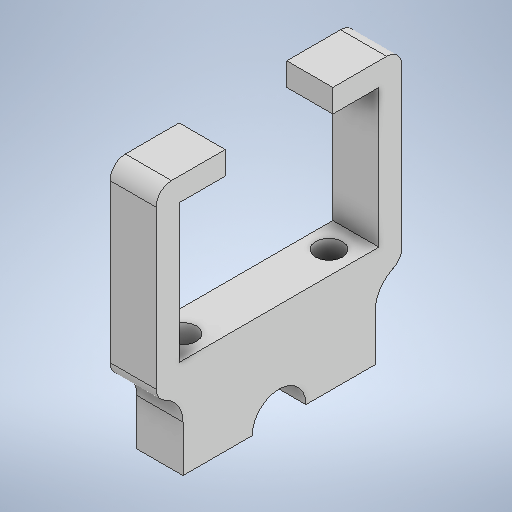
# Autodesk Inventor part: Base
Saved by Autodesk Inventor 2025 (Build 290162000, 162)
## iProperties
Created: 2024-06-05
Part Number: Base
Material: Générique
Document SubType Name: Modeling
Designer: luc4s
Density: 1 g/cm^3
Appearance: Par défaut
Author: luc4s
## iProperties of the stored document Bras_1_Impression 3D.ipt
Created: 2024-06-05
Part Number: Bras_1_Impression 3D
Material: Générique
Document SubType Name: Modeling
Designer: luc4s
Density: 1 g/cm^3
Appearance: Par défaut
Author: luc4s
Autodesk Inventor part; units mm, degrees
ref_plane "YZ Plane" through (0, 0, 0) normal (1, 0, 0) x (0, 1, 0)
ref_plane "XZ Plane" through (0, 0, 0) normal (0, 1, 0) x (-1, 0, 0)
ref_plane "XY Plane" through (0, 0, 0) normal (0, 0, 1) x (1, 0, 0)
sketch "Esquisse1" plane through (0, 0, 0) normal (1, 0, 0) x (0, 1, 0)
  arc A0 (0, -3.5) -> (0, 3.5) centre (0, 0) ccw
  line L0 (0, 6.2947) -> (0, -6.5718) construction
  line L1 (0, 3.5) -> (0, 12.5)
  line L2 (0, 12.5) -> (10, 12.5)
  line L3 (10, -12.5) -> (0, -12.5)
  line L4 (0, -12.5) -> (0, -3.5)
  line L5 (10, 12.5) -> (10, 16)
  line L6 (10, 16) -> (34, 16)
  line L7 (34, 16) -> (34, 7)
  line L8 (34, 7) -> (31, 7)
  line L9 (31, 7) -> (31, 13)
  line L10 (31, 13) -> (13, 13)
  line L11 (13, 13) -> (13, -13)
  line L12 (13, -13) -> (31, -13)
  line L13 (31, -13) -> (31, -7)
  line L14 (31, -7) -> (34, -7)
  line L15 (34, -7) -> (34, -16)
  line L16 (34, -16) -> (10, -16)
  line L17 (10, -16) -> (10, -12.5)
  point P0 (22, 13)
  dimension "d16" = 3.5
  dimension "d17" = 25
  dimension "d18" = 26
  dimension "d19" = 6
  dimension "d20" = 3
  dimension "d21" = 3
  dimension "d22" = 3
  dimension "d23" = 18
  dimension "d24" = 3
  dimension "d25" = 10
  constraints: 36 end point, 11 perpendicular, 10 point on line, 4 equal length, 2 point on circle, 2 vertical, 1 centre point, 1 coincident, 1 collinear, 1 midpoint
  measures "d16" radius of A0
  measures "d17" distance of L3.end L1.end
  measures "d18" distance of L10.end L11.end
  measures "d19" distance of L8.end L9.end
  measures "d20" distance from line of L6 point (22, 13)
  measures "d21" distance between parallel lines of L16 L12
  measures "d22" distance between parallel lines of L11 L5
  measures "d23" distance between parallel lines of L9 L11
  measures "d24" distance between parallel lines of L9 L7
  measures "d25" distance from line of L1.end L5
extrude "Extrusion1" add sketch "Esquisse1" along normal blind 6
fillet "Congé1" radius 4 2 edges at (3, 10, 12.5) (3, 10, -12.5)
fillet "Congé2" radius 2 2 edges at (3, 10, -16) (3, 10, 16)
fillet "Congé3" radius 2 2 edges at (3, 34, 16) (3, 34, -16)
sketch "Esquisse2" plane through (0, 0, -12.5) normal (0, -1, 0) x (1, 0, 0)
  circle A0 centre (3, 3) radius 1.75
  line L0 (0, -1.5) -> (0, 5.5) projected
  line L1 (6, -0.5) -> (6, 25.5) projected
  line L2 (0, -0.5) -> (0, 25.5) projected
  line L3 (0, 0) -> (6, 0) projected
  point P0 (0, 12.5)
  point P1 (3, 3)
  dimension "d28" = 3.5
  dimension "d31" = 3
  dimension "d32" = 3
  constraints: 1 centre point, 1 coincident
  measures "d28" diameter of A0
  measures "d31" distance from line of L3 point (3, 3)
  measures "d32" distance from line of L1 A0.centre
extrude "Extrusion2" cut sketch "Esquisse2" against normal blind 15
mirror "Mise en miroir1" about plane through (0, 0, 0) normal (0, 0, 1) of "Extrusion2"
